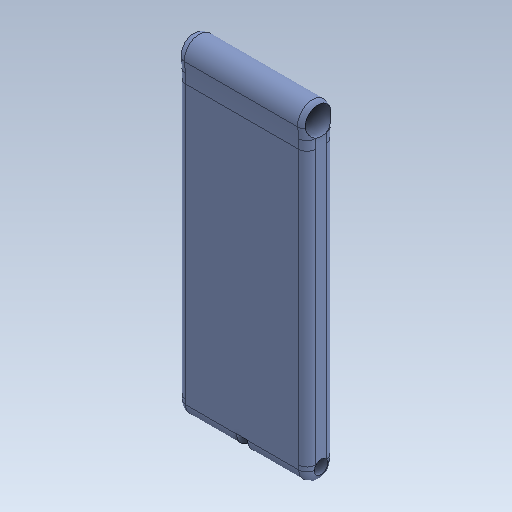
# Autodesk Inventor part: Top Watch Strap
Saved by Autodesk Inventor 2020 (Build 240168000, 168)
## iProperties
Created: 2020-05-08
Part Number: Top Watch Strap
Material: Rubber
Document SubType Name: Modeling
Designer: harry
Density: 0.93 g/cm^3
Appearance: Rubber - Blue
Author: harry
Autodesk Inventor part; units mm, degrees
ref_plane "YZ Plane" through (0, 0, 0) normal (1, 0, 0) x (0, 1, 0)
ref_plane "XZ Plane" through (0, 0, 0) normal (0, 1, 0) x (-1, 0, 0)
ref_plane "XY Plane" through (0, 0, 0) normal (0, 0, 1) x (1, 0, 0)
sketch "Sketch3" plane through (0, 0, 0) normal (1, 0, 0) x (0, 1, 0)
  circle A0 centre (0, 0) radius 3.5
  dimension "d6" = 7
  constraints: 1 centre point, 1 coincident
  measures "d6" diameter of A0
extrude "Extrusion2" add sketch "Sketch3" along normal mid plane 30.5
sketch "Sketch4" plane through (0, 0, 0) normal (1, 0, 0) x (0, 1, 0)
  line L0 (-70, 3.25) -> (-5, 3.25)
  line L1 (-5, 3.25) -> (-5, -3.25)
  line L2 (-5, -3.25) -> (-70, -3.25)
  line L3 (-70, -3.25) -> (-70, 3.25)
  line L4 (-70, 3.25) -> (-5, -3.25) construction
  line L5 (-5, 3.25) -> (-70, -3.25) construction
  circle A0 centre (0, 0) radius 3.5
  arc A1 (-5, 3.25) -> (-0.349127, 3.482544) centre (-5, 49.875) ccw
  arc A2 (-0.349127, -3.482544) -> (-5, -3.25) centre (-5, -49.875) ccw
  point P0 (-37.5, 0)
  point P1 (-37.5, 0)
  dimension "d9" = 6.5
  dimension "d12" = 70
  dimension "d13" = 5
  constraints: 12 end point, 6 point on circle, 4 tangent, 3 midpoint, 2 centre point, 2 parallel, 1 horizontal, 1 horizontal alignment, 1 perpendicular
  measures "d9" distance between parallel lines of L2 L0
  measures "d12" distance from line of point (0, 0) L3
  measures "d13" distance from line of L1 point (0, 0)
extrude "Extrusion3" add sketch "Sketch4" along normal mid plane 30.5 contours L0 L1 L2 L3 | A1 A0 A2 L1
sketch "Sketch8" plane through (15.25, 0, 0) normal (1, 0, 0) x (0, 0, -1)
  arc A0 (3.482544, -0.349127) -> (-3.482544, -0.349127) centre (0, 0) ccw
  constraints: 1 coincident
hole "Hole1" at (15.25, 0, 0) direction (-1, 0, 0) diameter 6.1 end through all
sketch "Sketch9" plane through (0, 0, 0) normal (1, 0, 0) x (0, 1, 0)
  line L0 (-70, -3.25) -> (-70, 3.25) projected
  circle A0 centre (-70, 0) radius 3.25
  point P0 (0, 0)
  constraints: 1 midpoint, 3 other
extrude "Extrusion7" add sketch "Sketch9" along normal mid plane 30.5 contours A0 L0 picked at (-71.075435, -0.130581)
sketch "Sketch10" plane through (0, 0, 0) normal (0, 0, 1) x (1, 0, 0)
  line L0 (-1.3, -70) -> (1.3, -70)
  line L1 (1.3, -70) -> (1.3, -73.25)
  line L2 (1.3, -73.25) -> (-1.3, -73.25)
  line L3 (-1.3, -73.25) -> (-1.3, -70)
  line L4 (-15.25, -70) -> (-15.25, -73.25)
  line L5 (-15.25, -0.349127) -> (15.25, -0.349127)
  line L6 (-21.35, 0) -> (21.35, 0)
  point P0 (0, -73.25)
  point P1 (0, -73.25)
  point P2 (0, -70)
  point P3 (0, -0.349127)
  dimension "d44" = 2.6
  dimension "d46" = 3.25
  constraints: 8 end point, 3 midpoint, 2 parallel, 1 coincident, 1 horizontal, 1 horizontal alignment, 1 perpendicular, 1 vertical alignment
  measures "d44" distance of L0.start L0.end
  measures "d46" distance of L2.end L0.start
revolve "Revolution1" cut sketch "Sketch10" angle 180 mid plane about axis through (-10, 0, 0) along (1, 0, 0)
sketch "Sketch11" plane through (15.25, 0, 0) normal (1, 0, 0) x (0, 0, -1)
  arc A0 (-3.25, -70) -> (3.25, -70) centre (0, -70) ccw projected
  point P0 (0, 0)
  constraints: 1 coincident
hole "Hole2" at (15.25, -70, 0) direction (-1, 0, 0) diameter 3.2 end through all
fillet "Fillet2" radius 2 12 edges at (15.25, -73.25, 0) (15.25, -37.5, -3.25) (15.25, -2.6717, -3.3082) (15.25, 3.5, 0) (15.25, -2.6717, 3.3082) (15.25, -37.5, 3.25) (-15.25, -2.6717, 3.3082) (-15.25, 3.5, 0) (-15.25, -2.6717, -3.3082) (-15.25, -37.5, -3.25) (-15.25, -73.25, 0) (-15.25, -37.5, 3.25)
body "Solid2"
